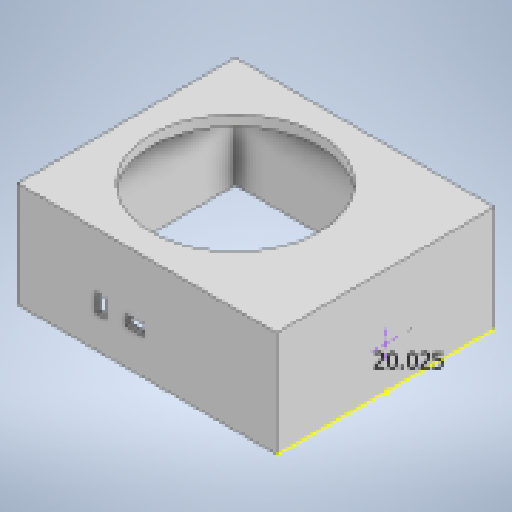
# Autodesk Inventor part: Bottom_Cover
Saved by Autodesk Inventor 2024 (Build 280153000, 153)
## iProperties
Created: 2023-12-19
Part Number: Bottom_Cover
Material: Generic
Document SubType Name: Modeling
Designer: 박동준
Density: 1 g/cm^3
Appearance: Default
Author: 박동준
Autodesk Inventor part; units mm, degrees
ref_plane "YZ Plane" through (0, 0, 0) normal (1, 0, 0) x (0, 1, 0)
ref_plane "XZ Plane" through (0, 0, 0) normal (0, 1, 0) x (-1, 0, 0)
ref_plane "XY Plane" through (0, 0, 0) normal (0, 0, 1) x (1, 0, 0)
sketch "Sketch1" plane through (0, 0, 0) normal (0, 1, 0) x (-1, 0, 0)
  line L0 (63, -53) -> (-63, -53)
  line L1 (-63, -53) -> (-63, 53)
  line L2 (-63, 53) -> (63, 53)
  line L3 (63, 53) -> (63, -53)
  point P0 (0, 0)
  point P1 (63, 0)
  point P2 (0, -53)
  dimension "d0" = 126
  dimension "d1" = 106
  constraints: 8 end point, 2 midpoint, 2 parallel, 1 horizontal, 1 horizontal alignment, 1 perpendicular, 1 vertical alignment
  measures "d0" distance of L1.end L2.end
  measures "d1" distance of L0.end L1.end
extrude "Extrusion1" add sketch "Sketch1" along normal blind 51.3
sketch "Sketch2" plane through (0, 0, 0) normal (0, -1, 0) x (1, 0, 0)
  line L0 (60.5, 50.5) -> (-60.5, 50.5)
  line L1 (-60.5, 50.5) -> (-60.5, -50.5)
  line L2 (-60.5, -50.5) -> (60.5, -50.5)
  line L3 (60.5, -50.5) -> (60.5, 50.5)
  line L4 (63, 53) -> (63, -53) projected
  line L5 (-63, 53) -> (63, 53) projected
  point P0 (0, 0)
  point P1 (60.5, 0)
  point P2 (0, 50.5)
  dimension "d8" = 2.5
  dimension "d9" = 2.5
  constraints: 8 end point, 2 midpoint, 2 parallel, 1 horizontal, 1 horizontal alignment, 1 perpendicular, 1 vertical alignment
  measures "d8" distance between parallel lines of L3 L4
  measures "d9" distance between parallel lines of L5 L0
extrude "Extrusion2" cut sketch "Sketch2" against normal blind 46.3
sketch "Sketch3" plane through (0, 51.3, 0) normal (0, 1, 0) x (1, 0, 0)
  circle A0 centre (-10.05, 0) radius 41
  line L0 (63, -53) -> (63, 53) projected
  point P0 (0, 0)
  point P1 (63, 0)
  dimension "d12" = 82
  dimension "d13" = 73.05
  constraints: 1 centre point, 1 horizontal alignment, 1 midpoint
  measures "d12" diameter of A0
  measures "d13" distance from line of A0.centre L0
extrude "Extrusion3" cut sketch "Sketch3" against normal blind 46.3
sketch "Sketch4" plane through (-63, 0, 53) normal (0, 0, 1) x (1, 0, 0)
  line L0 (37.95, 24.425) -> (42.95, 24.425)
  line L1 (42.95, 24.425) -> (42.95, 15.625)
  line L2 (42.95, 15.625) -> (37.95, 15.625)
  line L3 (37.95, 15.625) -> (37.95, 24.425)
  line L4 (0, 0) -> (126, 0) projected
  line L5 (0, 0) -> (0, 51.3) projected
  line L6 (52.95, 22.525) -> (61.75, 22.525)
  line L7 (61.75, 22.525) -> (61.75, 17.525)
  line L8 (61.75, 17.525) -> (52.95, 17.525)
  line L9 (52.95, 17.525) -> (52.95, 22.525)
  point P0 (63, 0)
  point P1 (57.35, 17.525)
  point P2 (40.45, 15.625)
  point P3 (42.95, 20.025)
  point P4 (52.95, 20.025)
  dimension "d16" = 5
  dimension "d17" = 8.8
  dimension "d18" = 15.625
  dimension "d19" = 37.95
  dimension "d20" = 8.8
  dimension "d21" = 5
  dimension "d22" = 10
  constraints: 16 end point, 4 midpoint, 4 parallel, 2 horizontal, 2 perpendicular, 1 horizontal alignment
  measures "d16" distance of L1.end L2.end
  measures "d17" distance of L0.end L1.end
  measures "d18" distance between parallel lines of L2 L4
  measures "d19" distance between parallel lines of L5 L3
  measures "d20" distance of L7.end L8.end
  measures "d21" distance of L6.end L7.end
  measures "d22" distance between parallel lines of L9 L1
extrude "Extrusion4" cut sketch "Sketch4" against normal blind 10
sketch "Sketch5" plane through (63, 0, 53) normal (1, 0, 0) x (0, 0, -1)
  line L0 (0, 0) -> (106, 0) projected
  line L1 (0, 51.3) -> (106, 51.3) projected
  circle A0 centre (53, 20.025) radius 2.15
  point P0 (53, 0)
  point P1 (53, 51.3)
  point P2 (53, 0)
  dimension "d26" = 4.3
  dimension "d27" = 20.025
  constraints: 2 midpoint, 1 centre point, 1 vertical alignment
  measures "d26" diameter of A0
  measures "d27" distance from line of L0 A0.centre
extrude "Extrusion5" cut sketch "Sketch5" against normal through all
equation "\"d20\" = d17"
equation "\"d21\" = d16"
body "Solid1"
